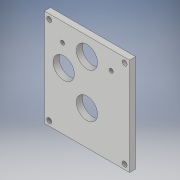
# Autodesk Inventor part: Gearbox Plate V2
Saved by Autodesk Inventor 2018 (Build 220112000, 112)
## iProperties
Created: 2019-01-19
Part Number: Gearbox Plate V2
Material: Generic
Document SubType Name: Modeling
Designer: maste
Density: 1 g/cm^3
Appearance: Default
Author: maste
Autodesk Inventor part; units mm, degrees
ref_plane "YZ Plane" through (0, 0, 0) normal (1, 0, 0) x (0, 1, 0)
ref_plane "XZ Plane" through (0, 0, 0) normal (0, 1, 0) x (-1, 0, 0)
ref_plane "XY Plane" through (0, 0, 0) normal (0, 0, 1) x (1, 0, 0)
sketch "Sketch1" plane through (0, 0, 0) normal (0, 0, 1) x (1, 0, 0)
  circle A0 centre (0, 0) radius 11.1125
  line L0 (0, 0) -> (-24.2467, 24.2467) construction
  line L1 (0, 0) -> (34.29, 0) construction
  circle A1 centre (-24.2467, 24.2467) radius 11.1125
  line L2 (-24.2467, 24.2467) -> (8.7733, 24.2467) construction
  line L3 (-24.2467, 24.2467) -> (0, 24.2467) construction
  line L4 (0, 24.2467) -> (0, 46.6502) construction
  line L5 (0, 46.6502) -> (-24.2467, 24.2467) construction
  circle A2 centre (0, 46.6502) radius 11.1125
  line L6 (0, 46.6502) -> (-25.4, 46.6502) construction
  line L7 (-25.4, 46.6502) -> (25.4, 46.6502) construction
  circle A3 centre (-25.4, 46.6502) radius 2.032
  circle A4 centre (25.4, 46.6502) radius 2.032
  line L8 (0, 46.6502) -> (0, 65.7002) construction
  line L9 (0, 65.7002) -> (44.45, 65.7002)
  line L10 (44.45, 65.7002) -> (44.45, -35.8998)
  line L11 (0, 65.7002) -> (-44.45, 65.7002)
  line L12 (-44.45, 65.7002) -> (-44.45, -35.8998)
  line L13 (-44.45, -35.8998) -> (44.45, -35.8998)
  dimension "d0" = 22.225
  dimension "d1" = 34.29
  dimension "d2" = 135
  dimension "d3" = 22.225
  dimension "d7" = 22.4035
  dimension "d8" = 22.225
  dimension "d9" = 25.4
  dimension "d10" = 50.8
  dimension "d11" = 4.064
  dimension "d12" = 19.05
  dimension "d13" = 101.6
  dimension "d14" = 44.45
  dimension "d17" = 44.45
  constraints: 28 end point, 5 centre point, 5 coincident, 5 perpendicular, 4 horizontal, 2 point on line, 1 equal length, 1 vertical
  measures "d0" diameter of A0
  measures "d1" distance of L0.start L0.end
  measures "d2" angle of L1 L0
  measures "d3" diameter of A1
  measures "d7" distance of L3.end L4.end
  measures "d8" diameter of A2
  measures "d9" distance of L6.start L6.end
  measures "d10" distance of L6.end L7.end
  measures "d11" diameter of A3
  measures "d12" distance of L6.start L8.end
  measures "d13" distance of L9.end L10.end
  measures "d14" distance of L8.end L11.end
  measures "d17" distance of L8.end L9.end
extrude "Extrusion1" add sketch "Sketch1" along normal blind 6.35
sketch "Sketch2" plane through (0, 0, 6.35) normal (0, 0, 1) x (1, 0, 0)
  line L0 (-44.45, 65.7002) -> (-39.37, 65.7002) construction
  line L1 (-44.45, 65.7002) -> (44.45, 65.7002) construction
  line L2 (-39.37, 65.7002) -> (-39.37, 60.6202) construction
  circle A0 centre (-39.37, 60.6202) radius 2.5797
  line L3 (0, 65.7002) -> (0, -35.8998) construction
  line L4 (-44.45, -35.8998) -> (44.45, -35.8998) construction
  line L5 (44.45, -35.8998) -> (44.45, 65.7002) construction
  line L6 (44.45, 14.9002) -> (-44.45, 14.9002) construction
  circle A1 centre (39.37, 60.6202) radius 2.5797
  circle A2 centre (-39.37, -30.8198) radius 2.5797
  circle A3 centre (39.37, -30.8198) radius 2.5797
  point P0 (0, 0)
  dimension "d18" = 5.08
  dimension "d19" = 5.08
  dimension "d20" = 5.1594
  constraints: 8 end point, 4 centre point, 3 midpoint, 3 symmetric about line, 1 coincident, 1 horizontal, 1 point on line, 1 vertical, 3 other
  measures "d18" distance of L0.start L0.end
  measures "d19" distance of L0.end L2.end
  measures "d20" diameter of A0
extrude "Extrusion2" cut sketch "Sketch2" against normal blind 25.4
body "Solid1"
